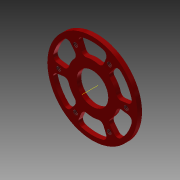
# Autodesk Inventor part: Carriage Plate - Gear Cover
Saved by Autodesk Inventor 2013 (Build 170138000, 138)
## iProperties
Created: 2013-04-01
Part Number: Carriage Plate - Gear Cover
Material: Generic
Document SubType Name: Sheet Metal
Designer: mvarma
Density: 1 g/cm^3
Sheet Metal Rule: Default
Author: mvarma
Autodesk Inventor part; units mm, degrees
ref_plane "YZ Plane" through (0, 0, 0) normal (1, 0, 0) x (0, 1, 0)
ref_plane "XZ Plane" through (0, 0, 0) normal (0, 1, 0) x (-1, 0, 0)
ref_plane "XY Plane" through (0, 0, 0) normal (0, 0, 1) x (1, 0, 0)
sketch "Sketch1" plane through (0, 0, 0) normal (0, 0, 1) x (1, 0, 0)
  circle A0 centre (0, 0) radius 23.8125 construction
  circle A1 centre (0, 0) radius 31.75
  line L0 (0, 0) -> (0, 23.8125) construction
  line L1 (-11.9062, 20.6222) -> (0, 0) construction
  circle A2 centre (0, 0) radius 11.1125
  circle A3 centre (0, 0) radius 28.575
  circle A4 centre (0, 0) radius 17.4625
  line L2 (-10.9352, 26.3999) -> (-6.6826, 16.1332)
  line L3 (0, 0) -> (-10.6305, 13.8539) construction
  line L4 (-10.6305, 13.8539) -> (-17.3954, 22.6701)
  line L5 (-6.6826, 16.1332) -> (0, 0) construction
  dimension "d0" = 47.625
  dimension "d1" = 63.5
  dimension "d2" = 30
  dimension "d15" = 22.225
  dimension "d16" = 57.15
  dimension "d17" = 34.925
  dimension "d18" = 7.5
  dimension "d19" = 7.5
  constraints: 12 end point, 6 point on circle, 5 centre point, 5 coincident, 2 collinear, 1 vertical
  measures "d0" diameter of A0
  measures "d1" diameter of A1
  measures "d2" angle of L0 L1
  measures "d15" diameter of A2
  measures "d16" diameter of A3
  measures "d17" diameter of A4
  measures "d18" angle of L1 L3
  measures "d19" angle of L2 L1
extrude "Plate2" add sketch "Sketch1" along normal blind 3.175 contours A1 | A4
sheet face with bend "Face3" sketch "Sketch1" thickness 3.175 toward (0, 0, 1) bend radius 3.175 relief tear relief width 3.175 relief depth 1.5875 picked at (-10.731, 22.4119) contours L2 A4 L4 A3
bend "Bend1"
hole "Hole2" at (-11.9062, 20.6222, 0) direction (0, 0, 1) diameter 3.302 end through all thread size "8-32 UNC" class "2B" standard "ANSI Unified Screw Threads"
fillet "Fillet1" radius 3.175 4 edges at (-17.3954, 22.6701, 1.5875) (-10.6305, 13.8539, 1.5875) (-6.6826, 16.1332, 1.5875) (-10.9352, 26.3999, 1.5875)
pattern_circular "Circular Pattern1" count 6 over 360 about axis through (0, 0, 0) along (0, 0, 1) of "Face3", "Hole2", "Fillet1"
equation "\"d31\" = Thickness"
equation "\"d21\" = BendRadius"
equation "\"d22\" = BendReliefWidth"
equation "\"d24\" = MinimumRemnant"
equation "\"d23\" = BendReliefDepth"
equation "\"d25\" = BendRadius"
equation "\"BendRadius\" = Thickness"
equation "\"BendReliefWidth\" = Thickness"
equation "\"BendReliefDepth\" = 0.5 * Thickness"
equation "\"CornerReliefSize\" = 4 * Thickness"
equation "\"MinimumRemnant\" = 2 * Thickness"
equation "\"TransitionRadius\" = BendRadius"
equation "\"JacobiRadiusSize\" = Thickness"
equation "\"GapSize\" = Thickness"
equation "\"d7\" = BendRadius"
equation "\"d20\" = BendRadius"
equation "\"Thickness\" = 3.175"
body "Solid2"
